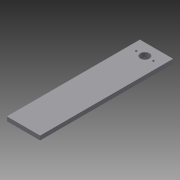
# Autodesk Inventor part: LowerArm
Saved by Autodesk Inventor 2013 (Build 170138000, 138)
## iProperties
Created: 2013-04-21
Part Number: LowerArm
Material: Generic
Document SubType Name: Modeling
Designer: fuji
Density: 1 g/cm^3
Author: fuji
Autodesk Inventor part; units mm, degrees
ref_plane "YZ Plane" through (0, 0, 0) normal (1, 0, 0) x (0, 1, 0)
ref_plane "XZ Plane" through (0, 0, 0) normal (0, 1, 0) x (-1, 0, 0)
ref_plane "XY Plane" through (0, 0, 0) normal (0, 0, 1) x (1, 0, 0)
sketch "Sketch2" plane through (0, 0, 0) normal (0, 1, 0) x (-1, 0, 0)
  line L0 (0, 0) -> (25.4, 0)
  line L1 (25.4, 0) -> (25.4, 101.6)
  line L2 (25.4, 101.6) -> (0, 101.6)
  line L3 (0, 101.6) -> (0, 0)
  circle A0 centre (12.7, 8.89) radius 3.5052
  circle A1 centre (6.1214, 8.89) radius 0.762
  circle A2 centre (19.2786, 8.89) radius 0.762
  dimension "d23" = 25.4
  dimension "d24" = 101.6
  dimension "d25" = 7.0104
  dimension "d26" = 8.89
  dimension "d27" = 12.7
  dimension "d28" = 1.524
  dimension "d29" = 1.524
  dimension "d30" = 13.1572
  dimension "d31" = 6.5786
  dimension "d32" = 8.89
  dimension "d33" = 8.89
  constraints: 8 end point, 3 centre point, 2 parallel, 1 horizontal, 1 perpendicular
  measures "d23" distance of L2.end L1.end
  measures "d24" distance of L1.end L0.end
  measures "d25" diameter of A0
  measures "d26" distance from line of A0.centre L0
  measures "d27" distance from line of A0.centre L3
  measures "d28" diameter of A1
  measures "d29" diameter of A2
  measures "d30" distance of A2.centre A1.centre
  measures "d31" distance of A0.centre A1.centre
  measures "d32" distance from line of A1.centre L0
  measures "d33" distance from line of A2.centre L0
extrude "Extrusion2" add sketch "Sketch2" along normal blind 3.175
equation "\"d23\" = d34"
equation "\"d24\" = d35"
equation "\"d25\" = d36"
equation "\"d26\" = d37"
equation "\"d27\" = 0.5 * d34"
equation "\"d28\" = d38"
equation "\"d29\" = d38"
equation "\"d30\" = d39"
equation "\"d31\" = 0.5 * d39"
equation "\"d32\" = d37"
equation "\"d33\" = d37"
equation "\"d40\" = thick"
equation "\"thick\" = 3.175"
equation "\"hornCenter\" = 7.0104"
equation "\"hornDia\" = 13.1572"
equation "\"hornOffset\" = 8.89"
equation "\"hornHole\" = 1.778"
equation "\"servoWidth\" = 12"
equation "\"servoDist\" = 35"
equation "\"servoHole\" = 2.1082"
equation "\"servoOff\" = 8.89"
equation "\"armWidth\" = 25.4"
equation "\"armLength\" = 101.6"
equation "\"d34\" = 25.4"
equation "\"d35\" = 101.6"
equation "\"d36\" = 7.0104"
equation "\"d37\" = 8.89"
equation "\"d38\" = 1.524"
equation "\"d39\" = 13.1572"
body "Solid2"
